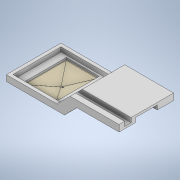
# Autodesk Inventor part: newconeholder
Saved by Autodesk Inventor 2021 (Build 250183000, 183)
## iProperties
Created: 2021-11-17
Part Number: newconeholder
Material: Generic
Document SubType Name: Modeling
Designer: mattc
Density: 1 g/cm^3
Appearance: Default
Author: mattc
Autodesk Inventor part; units mm, degrees
ref_plane "YZ Plane" through (0, 0, 0) normal (1, 0, 0) x (0, 1, 0)
ref_plane "XZ Plane" through (0, 0, 0) normal (0, 1, 0) x (-1, 0, 0)
ref_plane "XY Plane" through (0, 0, 0) normal (0, 0, 1) x (1, 0, 0)
sketch "cone top" plane through (0, 0, 0) normal (0, 1, 0) x (-1, 0, 0)
  line L0 (-7.5, 10) -> (7.5, 10)
  line L1 (7.5, 10) -> (7.5, -10)
  line L2 (7.5, -10) -> (-7.5, -10)
  line L3 (-7.5, -10) -> (-7.5, 10)
  line L4 (-7.5, 10) -> (7.5, -10) construction
  line L5 (7.5, 10) -> (-7.5, -10) construction
  point P0 (0, 0)
  dimension "d0" = 15
  dimension "d1" = 20
  constraints: 12 end point, 2 midpoint, 2 parallel, 1 horizontal, 1 perpendicular
  measures "d0" distance of L1.end L2.end
  measures "d1" distance of L0.end L1.end
ref_plane "Work Plane2" through (0, -2.25, 0) normal (0, 1, 0) x (-1, 0, 0)
sketch "fly slot" plane through (0, -2.25, 0) normal (0, 1, 0) x (-1, 0, 0)
  spline S0 degree 4 poles (0.3964, -0.0002) (0.3991, -0.0499) (0.4019, -0.1475) (0.3162, -0.3523) (0.1925, -0.3295) (-0.2287, -0.3672) (-0.6422, -0.361) (-1.2582, -0.0137) (-1.2268, -0.0002) knots 0 0 0 0 0 0.11031 0.216226 0.372169 0.55077 1 1 1 1 1
  line L0 (0.3964, -0.0002) -> (-1.2268, -0.0002)
  spline S1 degree 4 poles (0.3964, -0.0002) (0.3937, 0.0489) (0.3859, 0.145) (0.3272, 0.3535) (0.185, 0.3281) (-0.2182, 0.3684) (-0.6512, 0.3594) (-1.2552, 0.0138) (-1.2268, -0.0002) knots 0 0 0 0 0 0.11031 0.216226 0.372169 0.55077 1 1 1 1 1
  point P0 (0.3234, -0.2856)
  point P1 (0.2125, -0.337)
  point P2 (-0.4465, -0.3294)
  point P3 (-1.1043, -0.0852)
  point P4 (-0.0232, -0.3469)
  point P5 (0.3234, 0.2853)
  point P6 (0.2125, 0.3367)
  point P7 (-0.4465, 0.3291)
  point P8 (-1.1043, 0.0849)
  point P9 (-0.0232, 0.3466)
  constraints: 5 symmetric about line, 2 end point, 14 other
sketch "Sketch6" plane through (0, -2.25, 0) normal (0, 1, 0) x (-1, 0, 0)
  line L0 (-0.0165, -0.0313) -> (0.0165, -0.0313)
  line L1 (0.0165, -0.0313) -> (0.0165, 0.0313)
  line L2 (0.0165, 0.0313) -> (-0.0165, 0.0313)
  line L3 (-0.0165, 0.0313) -> (-0.0165, -0.0313)
  line L4 (-0.0165, -0.0313) -> (0.0165, 0.0313) construction
  line L5 (0.0165, -0.0313) -> (-0.0165, 0.0313) construction
  point P0 (0, 0)
  constraints: 12 end point, 2 midpoint, 2 parallel, 1 horizontal, 1 perpendicular
loft "Loft3" add profiles "cone top", "Sketch6"
shell "Shell1" thickness 0.1 removed faces 1 at (2.5, 0, 3.3333)
extrude "Extrusion4" cut sketch "fly slot" along normal blind 10
ref_plane "Work Plane3" through (-7.5, 0, 10) normal (0, 1, 0) x (1, 0, 0)
sketch "Sketch7" plane through (-7.5, 0, 10) normal (0, 1, 0) x (1, 0, 0)
  line L0 (20, 22.5) -> (-5, 22.5)
  line L1 (-5, 22.5) -> (-5, -2.5)
  line L2 (-5, -2.5) -> (20, -2.5)
  line L3 (20, -2.5) -> (20, 22.5)
  line L4 (20, 22.5) -> (-5, -2.5) construction
  line L5 (-5, 22.5) -> (20, -2.5) construction
  line L6 (15, 0) -> (7.7562, 9.6495) projected
  line L7 (0, 20) -> (15, 20)
  line L8 (15, 20) -> (15, 0)
  line L9 (15, 0) -> (0, 0)
  line L10 (0, 0) -> (0, 20)
  line L11 (0, 20) -> (15, 0) construction
  line L12 (15, 20) -> (0, 0) construction
  point P0 (7.5, 10)
  dimension "d32" = 25
  dimension "d33" = 25
  constraints: 24 end point, 4 midpoint, 4 parallel, 2 horizontal, 2 perpendicular
  measures "d32" distance of L2.end L1.end
  measures "d33" distance of L1.end L0.end
extrude "Extrusion5" add sketch "Sketch7" along normal blind 0.75
sketch "Sketch8" plane through (-7.5, 0.75, 10) normal (0, 1, 0) x (1, 0, 0)
  line L0 (-5, -2.5) -> (20, -2.5) projected
  line L1 (-5, 22.5) -> (20, 22.5)
  line L2 (20, 22.5) -> (20, -2.5)
  line L3 (20, -2.5) -> (-5, -2.5)
  line L4 (-5, -2.5) -> (-5, 22.5)
  line L5 (-5, 22.5) -> (20, -2.5) construction
  line L6 (20, 22.5) -> (-5, -2.5) construction
  line L7 (-3.5, 21) -> (18.5, 21)
  line L8 (18.5, 21) -> (18.5, -1)
  line L9 (18.5, -1) -> (-3.5, -1)
  line L10 (-3.5, -1) -> (-3.5, 21)
  line L11 (-3.5, 21) -> (18.5, -1) construction
  line L12 (18.5, 21) -> (-3.5, -1) construction
  point P0 (7.5, 10)
  dimension "d36" = 22
  dimension "d37" = 22
  constraints: 24 end point, 4 midpoint, 4 parallel, 2 horizontal, 2 perpendicular
  measures "d36" distance of L8.end L9.end
  measures "d37" distance of L7.end L8.end
extrude "Extrusion6" add sketch "Sketch8" along normal blind 2
move faces "Move1" translate (1.588, 0, 0) faces at (12.5, 1.8333, 4.1667)
sketch "Sketch9" plane through (-7.5, 2.75, 10) normal (0, 1, 0) x (1, 0, 0)
  line L0 (-5, -2.5) -> (21.588, -2.5) projected
  line L1 (21.588, 22.5) -> (18.5002, 22.5)
  line L2 (18.5002, 22.5) -> (18.5002, -2.5)
  line L3 (18.5002, -2.5) -> (21.588, -2.5)
  line L4 (21.588, -2.5) -> (21.588, 22.5)
  point P0 (7.5, 10)
  constraints: 8 end point, 2 parallel, 1 horizontal, 1 perpendicular, 1 point on line
extrude "Extrusion7" add sketch "Sketch9" along normal blind 6
sketch "Sketch10" plane through (14.088, 0, 12.5) normal (1, 0, 0) x (0, 0, -1)
  line L0 (0, 0) -> (0, 8.75) projected
  line L1 (25, 0) -> (25, 8.75) projected
  line L2 (0, 8.75) -> (25, 8.75)
  line L3 (25, 8.75) -> (25, 5.75)
  line L4 (25, 5.75) -> (0, 5.75)
  line L5 (0, 5.75) -> (0, 8.75)
  point P0 (12.5, 0)
  point P1 (0, 5.75)
  dimension "d45" = 3
  constraints: 8 end point, 2 parallel, 1 horizontal, 1 perpendicular, 1 point on line
  measures "d45" distance of L2.end L3.end
extrude "Extrusion8" add sketch "Sketch10" along normal blind 25
sketch "Sketch11" plane through (14.088, 5.75, -12.5) normal (0, -1, 0) x (1, 0, 0)
  line L0 (25, 0) -> (25, 25) projected
  line L1 (25, 7.5) -> (14, 7.5)
  line L2 (14, 7.5) -> (14, 17.5)
  line L3 (14, 17.5) -> (25, 17.5)
  line L4 (25, 17.5) -> (25, 7.5)
  point P0 (-14.088, 12.5)
  dimension "d48" = 11
  dimension "d49" = 10
  constraints: 8 end point, 2 parallel, 1 horizontal, 1 perpendicular, 1 point on line
  measures "d48" distance of L2.end L3.end
  measures "d49" distance of L1.end L2.end
extrude "Extrusion9" cut sketch "Sketch11" against normal blind 2
sketch "Sketch12" plane through (-7.5, 8.75, 10) normal (0, 1, 0) x (1, 0, 0)
  line L0 (46.588, -2.5) -> (46.588, 5) projected
  line L1 (46.588, 0.0025) -> (17.246, 0.0025)
  line L2 (17.246, 0.0025) -> (17.246, 3.0025)
  line L3 (17.246, 3.0025) -> (46.588, 3.0025)
  line L4 (46.588, 3.0025) -> (46.588, 0.0025)
  point P0 (7.5, 10)
  point P1 (46.588, 3.0025)
  dimension "d52" = 3
  constraints: 8 end point, 2 parallel, 1 horizontal, 1 perpendicular, 1 point on line
  measures "d52" distance of L1.end L2.end
extrude "Extrusion10" cut sketch "Sketch12" against normal blind 2
chamfer "Chamfer1" distance 5.7 angle 45 1 edges at (14.088, 5.75, 0)
chamfer "Chamfer2" distance 5.7 angle 45 1 edges at (11.0002, 8.75, -2.7513)
body "Solid4"
